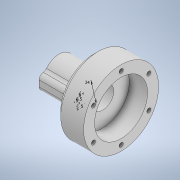
# Autodesk Inventor part: adapter
Saved by Autodesk Inventor 2020.3 (Build 243373000, 373)
## iProperties
Created: 2020-09-17
Part Number: adapter
Material: Generic
Document SubType Name: Modeling
Designer: joesp
Density: 1 g/cm^3
Appearance: Default
Author: joesp
Autodesk Inventor part; units mm, degrees
ref_plane "YZ Plane" through (0, 0, 0) normal (1, 0, 0) x (0, 1, 0)
ref_plane "XZ Plane" through (0, 0, 0) normal (0, 1, 0) x (-1, 0, 0)
ref_plane "XY Plane" through (0, 0, 0) normal (0, 0, 1) x (1, 0, 0)
sketch "Sketch1" plane through (0, 0, 0) normal (1, 0, 0) x (0, 1, 0)
  circle A0 centre (0, 0) radius 35 construction
  circle A1 centre (35, 0) radius 2.25
  circle A2 centre (-35, 0) radius 2.25
  circle A3 centre (17.5, -30.3109) radius 2.25
  circle A4 centre (-17.5, -30.3109) radius 2.25
  circle A5 centre (17.5, 30.3109) radius 2.25
  circle A6 centre (-17.5, 30.3109) radius 2.25
  circle A7 centre (0, 0) radius 29
  circle A8 centre (0, 0) radius 41
  dimension "d0" = 70
  dimension "d2" = 35
  dimension "d3" = 35
  dimension "d4" = 35
  dimension "d5" = 35
  dimension "d6" = 35
  dimension "d7" = 35
  dimension "d8" = 4.5
  dimension "d9" = 12
  dimension "d27" = 6
  constraints: 9 centre point, 6 point on circle, 5 equal radius, 3 coincident, 1 horizontal alignment
  measures "d0" diameter of A0
  measures "d2" distance of A1.centre A5.centre
  measures "d3" distance of A3.centre A1.centre
  measures "d4" distance of A4.centre A3.centre
  measures "d5" distance of A2.centre A4.centre
  measures "d6" distance of A6.centre A2.centre
  measures "d7" distance of A5.centre A6.centre
  measures "d8" diameter of A5
  measures "d9" radial gap between concentric circles of A8 A7
  measures "d27" radial gap between concentric circles of A0 A7
extrude "Extrusion1" add sketch "Sketch1" along normal blind 30
sketch "Sketch2" plane through (0, 0, 0) normal (-1, 0, 0) x (0, 0, 1)
  circle A0 centre (0, 0) radius 12
  line L0 (11.5515, 3.25) -> (16.5515, 3.25)
  line L1 (16.5515, 3.25) -> (16.5515, -3.25)
  line L2 (16.5515, -3.25) -> (11.5515, -3.25)
  line L3 (11.5515, -3.25) -> (11.5515, 3.25)
  circle A1 centre (0, 0) radius 17
  line L4 (14.864, 8.25) -> (21.5515, 8.25)
  line L5 (21.5515, 8.25) -> (21.5515, -8.25)
  line L6 (21.5515, -8.25) -> (14.864, -8.25)
  circle A2 centre (0, 0) radius 29
  circle A3 centre (0, 0) radius 29 projected
  point P0 (25, 0)
  dimension "d12" = 5
  dimension "d13" = 6.5
  dimension "d14" = 5
  dimension "d15" = 5
  dimension "d16" = 5
  dimension "d17" = 5
  dimension "d18" = 24
  constraints: 14 end point, 4 point on circle, 3 centre point, 3 coincident, 3 perpendicular, 2 horizontal, 2 parallel, 1 concentric
  measures "d12" distance of L0.start L0.end
  measures "d13" distance of L0.end L1.end
  measures "d14" distance between parallel lines of L0 L4
  measures "d15" distance between parallel lines of L5 L1
  measures "d16" distance between parallel lines of L2 L6
  measures "d17" radial gap between concentric circles of A1 A0
  measures "d18" diameter of A0
extrude "Extrusion2" add sketch "Sketch2" against normal blind 10 contours A1 | A1 L4 L5 L6 | A2
extrude "Extrusion3" add sketch "Sketch2" along normal blind 38 contours A1 | A1 L4 L5 L6
fillet "Fillet1" radius 5 4 edges at (-19, 8.25, 14.864) (-19, 8.25, 21.5515) (-19, -8.25, 21.5515) (-19, -8.25, 14.864)
chamfer "Chamfer1" distance 5 angle 45 7 edges at (0, 0, -17) (0, 8.8933, 15.1091) (0, 6.6533, 20.2614) (0, 0, 21.5515) (0, -6.6533, 20.2614) (0, -8.8933, 15.1091) (0, -41, 0)
equation "\"d2\" = d7"
equation "\"d3\" = d7"
equation "\"d4\" = d7"
equation "\"d5\" = d7"
equation "\"d6\" = d7"
equation "\"d27\" = 0.5 * d9"
body "Solid1"
